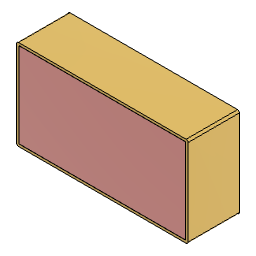
CronusPlastic (Autodesk Fusion 360 design; units mm, degrees)
Autodesk Fusion 360 part; units mm, degrees
note: some values were not read from the file. Chosen so that the rebuilt part matches the saved one: which face or edge a step refers to; which sketch regions a step uses.
sketch "Sketch1" plane through (0, 0, 0) normal (0, 1, 0) x (1, 0, 0) in component "Enclosure"
  line L0 (0, 0) -> (134.4, 0)
  line L1 (134.4, 0) -> (134.4, -70.6)
  line L2 (134.4, -70.6) -> (0, -70.6)
  line L3 (0, -70.6) -> (0, 0)
  dimension "d6" = 134.4
  dimension "d7" = 70.6
  constraint horizontal L0
  constraint vertical L1
  constraint horizontal L2
  constraint vertical L3
  constraint coincident L0.start L3.end
  measures "d6" distance of L0.start L0.end
  measures "d7" distance of L0.start L2.end
extrude "Extrude1" add sketch "Sketch1" along normal blind 40.3 makes body 1 in component "Enclosure"
shell "Shell1" thickness 3 removed faces 1 at (44.8, 0, 23.5333) on bodies 1 in component "Enclosure"
extrude "Extrude2" cut 1 faces at (45.8, 37.3, 24.5333) along direction (0, 1, 0) up to surface (3 mm away) on bodies 1 bodies 1 in component "Enclosure"
ref_plane "WorkPlane1" through (67.2, 2.4, 35.3) normal (0, -1, 0) x (-1, 0, 0) in component "Enclosure"
sketch "Sketch2" plane through (0, 0, 0) normal (0, -1, 0) x (1, 0, 0) in component "Enclosure"
  line L0 (3, 3) -> (3, 67.6)
  line L1 (3, 67.6) -> (131.4, 67.6)
  line L2 (131.4, 67.6) -> (131.4, 3)
  line L3 (131.4, 3) -> (3, 3)
  line L4 (134.4, 70.6) -> (0, 70.6)
  line L5 (0, 70.6) -> (0, 0)
  line L6 (0, 0) -> (134.4, 0)
  line L7 (134.4, 0) -> (134.4, 70.6)
  line L8 (132.4, 2) -> (2, 2)
  line L9 (2, 2) -> (2, 68.6)
  line L10 (2, 68.6) -> (132.4, 68.6)
  line L11 (132.4, 68.6) -> (132.4, 2)
  dimension "d15" = -1
extrude "Extrude3" cut sketch "Sketch2" against normal up to surface (2.4 mm away) contours L8 L9 L10 L11 bodies 1 in component "Enclosure"
sketch "Sketch1 (2)" plane through (0, 2.4, 0) normal (0, -1, 0) x (-1, 0, 0) in component "Display"
  line L0 (-131.4, -67.6) -> (-3, -67.6) construction
  line L1 (-131.4, -3) -> (-131.4, -67.6) construction
  line L2 (-3, -67.6) -> (-3, -3) construction
  line L3 (-3, -3) -> (-131.4, -3) construction
  line L4 (-131.2, -3.2) -> (-131.2, -67.4)
  line L5 (-131.2, -67.4) -> (-3.2, -67.4)
  line L6 (-3.2, -67.4) -> (-3.2, -3.2)
  line L7 (-3.2, -3.2) -> (-131.2, -3.2)
extrude "Extrude1'" add sketch "Sketch1 (2)" against normal blind 12.9 separate body makes body 2 in component "Display"
sketch "Sketch2 (2)" plane through (0, 15.3, 0) normal (0, 1, 0) x (-1, 0, 0) in component "Display"
  line L0 (-131.2, 67.4) -> (-131.2, 61.4) construction
  line L1 (-131.2, 61.4) -> (-3.2, 61.4) construction
  line L2 (-131.2, 61.4) -> (-128.2, 61.4) construction
  circle A0 centre (-128.2, 61.4) radius 1.65
  circle A1 centre (-96.2, 61.4) radius 1.65
  circle A2 centre (-64.2, 61.4) radius 1.65
  circle A3 centre (-32.2, 61.4) radius 1.65
  line L3 (-128.2, 61.4) -> (-102.2, 61.4) construction
  circle A4 centre (-102.2, 61.4) radius 1.65
  circle A5 centre (-70.2, 61.4) radius 1.65
  circle A6 centre (-38.2, 61.4) radius 1.65
  circle A7 centre (-6.2, 61.4) radius 1.65
  circle A8 centre (-128.2, 41.4) radius 1.65
  circle A9 centre (-96.2, 41.4) radius 1.65
  circle A10 centre (-64.2, 41.4) radius 1.65
  circle A11 centre (-32.2, 41.4) radius 1.65
  circle A12 centre (-102.2, 41.4) radius 1.65
  circle A13 centre (-70.2, 41.4) radius 1.65
  circle A14 centre (-38.2, 41.4) radius 1.65
  circle A15 centre (-6.2, 41.4) radius 1.65
  line L4 (-131.2, 35.3) -> (-3.2, 35.3) construction
  circle A16 centre (-128.2, 9.2) radius 1.65
  circle A17 centre (-128.2, 29.2) radius 1.65
  circle A18 centre (-102.2, 29.2) radius 1.65
  circle A19 centre (-102.2, 9.2) radius 1.65
  circle A20 centre (-96.2, 9.2) radius 1.65
  circle A21 centre (-96.2, 29.2) radius 1.65
  circle A22 centre (-70.2, 29.2) radius 1.65
  circle A23 centre (-70.2, 9.2) radius 1.65
  circle A24 centre (-64.2, 9.2) radius 1.65
  circle A25 centre (-64.2, 29.2) radius 1.65
  circle A26 centre (-38.2, 9.2) radius 1.65
  circle A27 centre (-32.2, 9.2) radius 1.65
  circle A28 centre (-38.2, 29.2) radius 1.65
  circle A29 centre (-32.2, 29.2) radius 1.65
  circle A30 centre (-6.2, 9.2) radius 1.65
  circle A31 centre (-6.2, 29.2) radius 1.65
  line L5 (-131.2, 3.2) -> (-3.2, 3.2)
  line L6 (-3.2, 3.2) -> (-3.2, 67.4)
  line L7 (-3.2, 67.4) -> (-131.2, 67.4)
  line L8 (-131.2, 67.4) -> (-131.2, 3.2)
  dimension "d20" = 6
  dimension "d21" = 3
  dimension "d22" = 3.3
  dimension "d25" = 32
  dimension "d26" = -20
  dimension "d27" = 26
  dimension "d28" = 3.3
  dimension "d31" = 32
  dimension "d32" = -20
  constraint perpendicular L0 L2
  constraint coincident L2.end A0.centre
  constraint parallel L1 L3
  constraint coincident L3.end A4.centre
  constraint symmetric A0 L4 A16
  constraint symmetric A1 L4 A20
  constraint symmetric A2 L4 A24
  constraint symmetric A3 L4 A27
  constraint symmetric A4 L4 A19
  constraint symmetric A5 L4 A23
  constraint symmetric A6 L4 A26
  constraint symmetric A7 L4 A30
  constraint symmetric A8 L4 A17
  constraint symmetric A9 L4 A21
  constraint symmetric A10 L4 A25
  constraint symmetric A11 L4 A29
  constraint symmetric A12 L4 A18
  constraint symmetric A13 L4 A22
  constraint symmetric A14 L4 A28
  constraint symmetric A15 L4 A31
  constraint coincident L1.end L6
  constraint coincident L0.end L8
  constraint coincident L0.start L7.end
  constraint midpoint L4.start L8
  constraint midpoint L4.end L6
  measures "d20" distance of L0.end L0.start
  measures "d21" distance of L0.end L2.end
  measures "d22" diameter of A0
  measures "d27" distance of L2.end L3.end
  measures "d28" diameter of A4
extrude "Extrude2'" cut sketch "Sketch2 (2)" against normal blind 2 contours A0 | A1 | A2 | A3 | A4 | A5 | A6 | A7 | A8 | A9 | A10 | A11 | A12 | A13 | A14 | A15 | A16 | A17 | A18 | A19 | A20 | A21 | A22 | A23 | A24 | A25 | A26 | A27 | A28 | A29 | A30 | A31 bodies 2 in component "Display"
sketch "Sketch1 (3)" plane through (0, 15.3, 0) normal (0, 1, 0) x (-1, 0, 0) in component "DisplayMount"
  line L0 (-67.2, 67.4) -> (-67.2, 3.2) construction
  line L1 (-131.2, 3.2) -> (-3.2, 3.2)
  line L2 (-3.2, 3.2) -> (-3.2, 67.4)
  line L3 (-3.2, 67.4) -> (-131.2, 67.4)
  line L4 (-131.2, 67.4) -> (-131.2, 3.2)
  line L5 (-131.2, 67.4) -> (-67.2, 67.4) construction
  line L6 (-99.2, 67.4) -> (-99.2, 3.2) construction
  line L7 (-92.7, 3.2) -> (-105.7, 3.2)
  line L8 (-105.7, 3.2) -> (-105.7, 67.4)
  line L9 (-105.7, 67.4) -> (-92.7, 67.4)
  line L10 (-92.7, 67.4) -> (-92.7, 3.2)
  line L11 (-92.7, 3.2) -> (-105.7, 67.4) construction
  line L12 (-105.7, 3.2) -> (-92.7, 67.4) construction
  line L13 (-28.7, 3.2) -> (-28.7, 67.4)
  line L14 (-28.7, 67.4) -> (-41.7, 67.4)
  line L15 (-41.7, 67.4) -> (-41.7, 3.2)
  line L16 (-41.7, 3.2) -> (-28.7, 3.2)
  line L17 (-105.7, 3.2) -> (-92.7, 3.2)
  line L18 (-92.7, 3.2) -> (-92.7, 6.2)
  line L19 (-92.7, 6.2) -> (-105.7, 6.2)
  line L20 (-105.7, 6.2) -> (-105.7, 3.2)
  line L21 (-41.7, 3.2) -> (-28.7, 3.2)
  line L22 (-28.7, 3.2) -> (-28.7, 6.2)
  line L23 (-28.7, 6.2) -> (-41.7, 6.2)
  line L24 (-41.7, 6.2) -> (-41.7, 3.2)
  circle A0 centre (-96.2, 61.4) radius 1.65
  circle A1 centre (-102.2, 41.4) radius 1.65
  circle A2 centre (-38.2, 61.4) radius 1.65
  circle A3 centre (-32.2, 41.4) radius 1.65
  circle A4 centre (-102.2, 29.2) radius 1.65
  circle A5 centre (-96.2, 9.2) radius 1.65
  circle A6 centre (-32.2, 29.2) radius 1.65
  circle A7 centre (-38.2, 9.2) radius 1.65
  line L25 (-105.7, 67.4) -> (-92.6, 67.4)
  line L26 (-92.6, 67.4) -> (-92.6, 64.4)
  line L27 (-92.6, 64.4) -> (-105.7, 64.4)
  line L28 (-105.7, 64.4) -> (-105.7, 67.4)
  line L29 (-41.7, 67.4) -> (-28.7, 67.4)
  line L30 (-28.7, 67.4) -> (-28.7, 64.4)
  line L31 (-28.7, 64.4) -> (-41.7, 64.4)
  line L32 (-41.7, 64.4) -> (-41.7, 67.4)
  point P0 (-99.2, 35.3)
  dimension "d58" = 13
  dimension "d59" = 3
  dimension "d60" = 3
  dimension "d92" = 3
  dimension "d93" = 3
  constraint midpoint L0.start L3
  constraint midpoint L0.end L1
  constraint coincident L3.end L4.start
  constraint midpoint L5 L6.start
  constraint perpendicular L1 L6
  constraint horizontal L7
  constraint perpendicular L7 L8
  constraint parallel L7 L9
  constraint parallel L8 L10
  constraint coincident L11 P0
  constraint coincident L12 P0
  constraint midpoint L6 P0
  constraint symmetric L0 L7.start L15.end
  constraint symmetric L0 L7.end L13.start
  constraint symmetric L0 L8.end L13.end
  constraint symmetric L0 L9.end L14.end
  constraint horizontal L17
  constraint vertical L18
  constraint horizontal L19
  constraint vertical L20
  constraint coincident L10 L18.end
  constraint horizontal L21
  constraint vertical L22
  constraint horizontal L23
  constraint vertical L24
  constraint coincident L13 L22.end
  constraint collinear L5 L9
  constraint collinear L1 L17
  constraint horizontal L25
  constraint vertical L26
  constraint horizontal L27
  constraint vertical L28
  constraint horizontal L29
  constraint vertical L30
  constraint horizontal L31
  constraint vertical L32
  constraint collinear L13 L30
  measures "d58" distance of L8.end L9.end
  measures "d59" distance of L7.end L19.end
  measures "d60" distance of L15.end L23.end
  measures "d92" distance of L8.end L27.end
  measures "d93" distance of L14.end L31.end
extrude "Extrude1''" add sketch "Sketch1 (3)" along normal blind 3 separate body contours L8 L10 L19 L27 | L3 L8 L9 L10 L25 L27 L28 | L13 L15 L23 L31 | L3 L13 L14 L15 L29 L30 L31 L32 makes body 3 at (101.9708, 15.3, 14.7288) makes body 4 at (32.4292, 15.3, 14.7288) in component "DisplayMount"
extrude "Extrude2''" add sketch "Sketch1 (3)" along normal blind 23.2 contours L1 L7 L8 L10 L17 L18 L19 L20 | L3 L8 L9 L10 L25 L27 L28 | L1 L13 L15 L16 L21 L22 L23 L24 | L3 L13 L14 L15 L29 L30 L31 L32 bodies 3 4 in component "DisplayMount"
chamfer "Chamfer1" distance 4 angle 45 2 edges at (99.2, 18.3, 6.2) (35.2, 18.3, 6.2) on bodies 3 4 in component "DisplayMount"
chamfer "Chamfer1" distance 4 angle 45 2 edges at (99.2, 18.3, 64.4) (35.2, 18.3, 64.4) on bodies 3 4 in component "DisplayMount"
sketch "Sketch3" plane through (0, 18.3, 0) normal (0, 1, 0) x (-1, 0, 0) in component "DisplayMount"
  line L0 (-105.7, 10.2) -> (-28.6, 67.9) construction
  line L1 (-67.15, 39.05) -> (-67.15, 35.65) construction
  line L2 (-34.15, 12.65) -> (-100.15, 12.65) construction
  line L3 (-100.15, 12.65) -> (-100.15, 58.65) construction
  line L4 (-100.15, 58.65) -> (-34.15, 58.65) construction
  line L5 (-34.15, 58.65) -> (-34.15, 12.65) construction
  line L6 (-34.15, 12.65) -> (-100.15, 58.65) construction
  line L7 (-100.15, 12.65) -> (-34.15, 58.65) construction
  circle A0 centre (-100.15, 58.65) radius 1
  circle A1 centre (-100.15, 58.65) radius 2.15
  circle A2 centre (-34.15, 58.65) radius 2.15
  circle A3 centre (-34.15, 58.65) radius 1
  circle A4 centre (-100.15, 12.65) radius 2.15
  circle A5 centre (-100.15, 12.65) radius 1
  circle A6 centre (-34.15, 12.65) radius 2.15
  circle A7 centre (-34.15, 12.65) radius 1
  circle A8 centre (-96.2, 61.4) radius 3
  circle A9 centre (-38.2, 61.4) radius 3
  circle A10 centre (-96.2, 9.2) radius 1.65
  circle A11 centre (-38.2, 9.2) radius 1.65
  circle A12 centre (-96.2, 9.2) radius 3
  circle A13 centre (-38.2, 9.2) radius 3
  arc A14 (-97.5124, 60.4) -> (-94.8876, 60.4) centre (-96.2, 61.4) ccw
  arc A15 (-39.5124, 60.4) -> (-36.8876, 60.4) centre (-38.2, 61.4) ccw
  point P0 (-105.7, 10.2)
  point P1 (-28.7, 67.4)
  dimension "d65" = 3.4
  dimension "d66" = 66
  dimension "d67" = 46
  dimension "d70" = 2
  dimension "d71" = 4.3
  dimension "d74" = 66
  dimension "d75" = -46
  dimension "d76" = 6
  dimension "d77" = 6
  dimension "d89" = 6
  dimension "d90" = 6
  constraint coincident P0 L0.start
  constraint vertical L1
  constraint midpoint L0 L1.start
  constraint horizontal L2
  constraint perpendicular L2 L3
  constraint parallel L2 L4
  constraint parallel L3 L5
  constraint coincident L3.end L4.start
  constraint concentric A0 A1
  constraint concentric A8 A14
  constraint concentric A9 A15
  constraint concentric A10 A12
  constraint concentric A11 A13
  constraint midpoint L1.end L7
  measures "d65" distance of L1.start L1.end
  measures "d66" distance of L3.end L4.end
  measures "d67" distance of L2.end L3.end
  measures "d70" diameter of A0
  measures "d71" diameter of A1
  measures "d76" diameter of A8
  measures "d77" diameter of A9
  measures "d89" diameter of A12
  measures "d90" diameter of A13
extrude "Extrude5" add sketch "Sketch3" along normal blind 4 contours A1 A8 | A1 A8 | A2 A9 | A2 A9 | A4 | A6 picked at (-99.3568, 60.1302) picked at (-98.5668, 59.7522) picked at (-35.7986, 59.0039) picked at (-35.8985, 59.6123) bodies 3 4 in component "DisplayMount"
chamfer "Chamfer2" distance 2 angle 45 4 edges at (100.15, 18.3, 56.5) (102.1545, 18.3, 13.4275) (34.15, 18.3, 56.5) (36.1545, 18.3, 13.4275) on bodies 3 4 in component "DisplayMount"
extrude "Extrude6" cut sketch "Sketch3" along normal up to surface (20.2 mm away) contours A1 A8 | A2 A9 | A12 | A13 picked at (-95.3701, 62.1374) picked at (-39.1425, 61.9294) bodies 3 4 in component "DisplayMount"
extrude "Extrude7" cut sketch "Sketch3" along normal up to surface (20.2 mm away) contours A1 A8 | A1 A8 | A2 A9 | A2 A9 | A3 | A12 | A13 picked at (-98.5668, 59.7522) picked at (-95.3701, 62.1374) picked at (-35.8985, 59.6123) picked at (-39.1425, 61.9294) bodies 3 4 in component "DisplayMount"
extrude "Extrude8" cut sketch "Sketch3" against normal up to surface (3 mm away) contours A0 | A3 | A5 | A7 bodies 3 4 in component "DisplayMount"
sketch "Sketch4" plane through (0, 38.5, 0) normal (0, 1, 0) x (-1, 0, 0) in component "DisplayMount"
  line L0 (-105.7, 67.4) -> (-102.518, 64.218) construction
  line L1 (-105.7, 67.4) -> (-99.6, 67.4) construction
  circle A0 centre (-102.518, 64.218) radius 1.5
  circle A1 centre (-102.518, 64.218) radius 2.95
  line L2 (-92.7, 67.4) -> (-41.7, 67.4) construction
  line L3 (-92.7, 3.2) -> (-41.7, 3.2) construction
  line L4 (-67.2, 67.4) -> (-67.2, 3.2) construction
  line L5 (-67.2, 35.3) -> (-57.2, 35.3) construction
  circle A2 centre (-31.882, 64.218) radius 2.95
  circle A3 centre (-31.882, 64.218) radius 1.5
  circle A4 centre (-102.518, 6.382) radius 2.95
  circle A5 centre (-102.518, 6.382) radius 1.5
  circle A6 centre (-31.882, 6.382) radius 2.95
  circle A7 centre (-31.882, 6.382) radius 1.5
  point P0 (-105.7, 67.4)
  point P1 (-92.7, 67.4)
  point P2 (-41.7, 67.4)
  point P3 (-92.7, 3.2)
  point P4 (-41.7, 3.2)
  dimension "d95" = 45
  dimension "d96" = 4.5
  dimension "d97" = 3
  dimension "d98" = 10
  dimension "d220" = 5.9
  constraint horizontal L1
  constraint coincident P0 L0.start
  constraint coincident L0.end A0.centre
  constraint concentric A0 A1
  constraint coincident P1 L2.start
  constraint coincident P2 L2.end
  constraint coincident P3 L3.start
  constraint coincident P4 L3.end
  constraint midpoint L2 L4.start
  constraint midpoint L3 L4.end
  constraint horizontal L5
  constraint midpoint L4 L5.start
  constraint symmetric A0 L4 A3
  constraint symmetric A1 L4 A2
  constraint symmetric A0 L5 A5
  constraint symmetric A1 L5 A4
  constraint symmetric L5 A2 A6
  constraint symmetric L5 A3 A7
  measures "d95" angle of L0 L1
  measures "d96" distance of P0 L0.end
  measures "d97" diameter of A0
  measures "d98" distance of L5.start L5.end
  measures "d220" diameter of A1
extrude "Extrude9" add sketch "Sketch4" against normal up to surface (23.2 mm away) bodies 3 4 in component "DisplayMount"
extrude "Extrude10" cut sketch "Sketch4" against normal up to surface (20.2 mm away) contours A0 | A3 | A5 | A7 bodies 3 4 in component "DisplayMount"
ref_plane "WorkPlane2" through (67.2, 38.5, 35.3) normal (0, 1, 0) x (0, 0, 1) in component "Enclosure"
sketch "Sketch5" plane through (0, 38.5, 0) normal (0, 1, 0) x (1, 0, 0) in component "Enclosure"
  line L0 (131.4, -3) -> (131.4, -67.6) construction
  line L1 (131.4, -67.6) -> (3, -67.6) construction
  line L2 (3, -3) -> (131.4, -3) construction
  line L3 (3, -67.6) -> (3, -3) construction
  line L4 (67.2, -67.6) -> (67.2, -3) construction
  line L5 (131.4, -35.3) -> (3, -35.3) construction
  line L6 (131.4, -3) -> (3, -3)
  line L7 (131.4, -3) -> (140.1172, -3) construction
  line L8 (129.9, -32.3) -> (132.9, -32.3)
  line L9 (132.9, -32.3) -> (132.9, -38.3)
  line L10 (132.9, -38.3) -> (129.9, -38.3)
  line L11 (129.9, -38.3) -> (129.9, -32.3)
  line L12 (129.9, -32.3) -> (132.9, -38.3) construction
  line L13 (132.9, -32.3) -> (129.9, -38.3) construction
  line L14 (1.5, -38.3) -> (4.5, -38.3)
  line L15 (4.5, -38.3) -> (4.5, -32.3)
  line L16 (4.5, -32.3) -> (1.5, -32.3)
  line L17 (131.4, -3) -> (131.4, -67.6)
  line L18 (131.4, -67.6) -> (3, -67.6)
  line L19 (3, -67.6) -> (3, -3)
  line L20 (3, -3) -> (131.4, -3)
  line L21 (0, -70.6) -> (134.4, -70.6)
  line L22 (134.4, -70.6) -> (134.4, 0)
  line L23 (134.4, 0) -> (0, 0)
  line L24 (0, 0) -> (0, -70.6)
  line L25 (131.4, -67.6) -> (126.4, -67.6)
  line L26 (126.4, -67.6) -> (126.4, -62.6)
  line L27 (126.4, -62.6) -> (131.4, -62.6)
  line L28 (131.4, -62.6) -> (131.4, -67.6)
  line L29 (126.4, -62.6) -> (131.4, -67.6) construction
  circle A0 centre (128.9, -65.1) radius 1.4
  line L30 (3, -67.6) -> (8, -67.6)
  line L31 (3, -62.6) -> (3, -67.6)
  circle A1 centre (5.5, -65.1) radius 1.4
  line L32 (8, -62.6) -> (3, -62.6)
  line L33 (8, -67.6) -> (8, -62.6)
  line L34 (126.4, -3) -> (126.4, -8)
  line L35 (126.4, -8) -> (131.4, -8)
  circle A2 centre (128.9, -5.5) radius 1.4
  line L36 (131.4, -8) -> (131.4, -3)
  line L37 (131.4, -3) -> (126.4, -3)
  line L38 (8, -3) -> (8, -8)
  line L39 (3, -3) -> (8, -3)
  circle A3 centre (5.5, -5.5) radius 1.4
  line L40 (8, -8) -> (3, -8)
  line L41 (3, -8) -> (3, -3)
  line L42 (105.7, -67.4) -> (105.7, -64.4) construction
  line L43 (92.7, -64.4) -> (92.7, -67.4) construction
  line L44 (131.4, -67.6) -> (3, -67.6) construction
  line L45 (108.7, -67.6) -> (105.7, -67.6)
  line L46 (105.7, -67.6) -> (105.7, -64.6)
  line L47 (105.7, -64.6) -> (108.7, -64.6)
  line L48 (108.7, -64.6) -> (108.7, -67.6)
  line L49 (92.7, -67.6) -> (89.7, -67.6)
  line L50 (89.7, -67.6) -> (89.7, -64.6)
  line L51 (89.7, -64.6) -> (92.7, -64.6)
  line L52 (92.7, -64.6) -> (92.7, -67.6)
  line L53 (25.7, -64.6) -> (25.7, -67.6)
  line L54 (25.7, -67.6) -> (28.7, -67.6)
  line L55 (28.7, -64.6) -> (25.7, -64.6)
  line L56 (28.7, -67.6) -> (28.7, -64.6)
  line L57 (44.7, -64.6) -> (41.7, -64.6)
  line L58 (41.7, -64.6) -> (41.7, -67.6)
  line L59 (44.7, -67.6) -> (44.7, -64.6)
  line L60 (41.7, -67.6) -> (44.7, -67.6)
  line L61 (105.7, -6) -> (108.7, -6)
  line L62 (108.7, -6) -> (108.7, -3)
  line L63 (108.7, -3) -> (105.7, -3)
  line L64 (105.7, -3) -> (105.7, -6)
  line L65 (92.7, -6) -> (92.7, -3)
  line L66 (89.7, -6) -> (92.7, -6)
  line L67 (89.7, -3) -> (89.7, -6)
  line L68 (92.7, -3) -> (89.7, -3)
  line L69 (44.7, -6) -> (41.7, -6)
  line L70 (44.7, -3) -> (44.7, -6)
  line L71 (41.7, -6) -> (41.7, -3)
  line L72 (41.7, -3) -> (44.7, -3)
  line L73 (28.7, -3) -> (28.7, -6)
  line L74 (25.7, -3) -> (28.7, -3)
  line L75 (28.7, -6) -> (25.7, -6)
  line L76 (25.7, -6) -> (25.7, -3)
  point P0 (131.4, -35.3)
  dimension "d110" = 3
  dimension "d111" = 6
  dimension "d183" = 5
  dimension "d184" = 5
  dimension "d185" = 2.8
  dimension "d199" = 3
  dimension "d200" = 3
  dimension "d201" = 3
  dimension "d202" = 3
  constraint midpoint L2 L4.end
  constraint midpoint L0 P0
  constraint midpoint L3 L5.end
  constraint horizontal L8
  constraint perpendicular L8 L9
  constraint parallel L8 L10
  constraint parallel L9 L11
  constraint coincident L12 P0
  constraint coincident L13 P0
  constraint coincident P0 L5.start
  constraint symmetric L4 L8.start L15.end
  constraint symmetric L4 L8.end L16.end
  constraint symmetric L4 L9.end L14.start
  constraint symmetric L4 L10.end L14.end
  constraint midpoint L1 L4.start
  constraint horizontal L25
  constraint vertical L26
  constraint horizontal L27
  constraint vertical L28
  constraint coincident L0.end L1.start
  constraint midpoint L29 A0.centre
  constraint symmetric L4 L0.end L1.end
  constraint symmetric L4 L25.end L30.end
  constraint symmetric L4 L26.end L32.start
  constraint symmetric L4 L27.end L31.start
  constraint symmetric L4 A0 A1
  constraint symmetric L5 L0.end L0.start
  constraint symmetric L5 L25.end L34.start
  constraint symmetric L5 L26.end L34.end
  constraint symmetric L5 L27.end L35.end
  constraint symmetric L5 A0 A2
  constraint symmetric L5 L1.end L2.start
  constraint symmetric L5 L30.end L38.start
  constraint symmetric L5 L31.start L40.end
  constraint symmetric L5 A1 A3
  constraint symmetric L5 L32.start L38.end
  constraint horizontal L45
  constraint vertical L46
  constraint horizontal L47
  constraint vertical L48
  constraint coincident L44 L45.start
  constraint collinear L42 L46
  constraint horizontal L49
  constraint vertical L50
  constraint horizontal L51
  constraint vertical L52
  constraint coincident L44 L49.start
  constraint collinear L43 L52
  constraint symmetric L4 L45.start L53.end
  constraint symmetric L4 L45.end L54.end
  constraint symmetric L4 L46.end L55.start
  constraint symmetric L4 L47.end L53.start
  constraint symmetric L4 L49.start L58.end
  constraint symmetric L4 L49.end L59.start
  constraint symmetric L4 L50.end L57.start
  constraint symmetric L4 L51.end L57.end
  constraint symmetric L5 L45.start L62.end
  constraint symmetric L5 L45.end L63.end
  constraint symmetric L5 L46.end L61.start
  constraint symmetric L5 L47.end L61.end
  constraint symmetric L5 L49.start L65.end
  constraint symmetric L5 L49.end L67.start
  constraint symmetric L5 L50.end L66.start
  constraint symmetric L5 L51.end L65.start
  constraint symmetric L5 L53.start L75.end
  constraint symmetric L5 L53.end L74.start
  constraint symmetric L5 L54.end L73.start
  constraint symmetric L5 L55.start L73.end
  constraint symmetric L5 L57.start L69.start
  constraint symmetric L5 L57.end L69.end
  constraint symmetric L5 L58.end L71.end
  constraint symmetric L5 L59.start L70.start
  measures "d110" distance of L9.end L10.end
  measures "d111" distance of L8.end L9.end
  measures "d183" distance of L0.end L25.end
  measures "d184" distance of L0.end L27.end
  measures "d185" diameter of A0
  measures "d199" distance of L45.start L45.end
  measures "d200" distance of L45.start L47.end
  measures "d201" distance of L49.start L49.end
  measures "d202" distance of L49.start L51.end
extrude "Extrude8'" add sketch "Sketch5" against normal blind 10 contours L6 L17 L20 L34 L35 L36 L37 | L17 L18 L25 L26 L27 L28 | L6 L19 L20 L38 L39 L40 L41 | L18 L19 L30 L31 L32 L33 | A0 | A1 | A2 | A3 bodies 1 in component "Enclosure"
extrude "Extrude19" add sketch "Sketch5" against normal blind 3 contours L8 L10 L11 L17 | L14 L15 L16 L19 bodies 1 in component "Enclosure"
extrude "Extrude14" cut sketch "Sketch5" against normal up to surface (9 mm away) contours A0 | A1 | A2 | A3 bodies 1 in component "Enclosure"
chamfer "Chamfer6" distance 4.9 angle 45 6 edges at (128.9, 28.5, 3) (128.9, 28.5, 67.6) (5.5, 28.5, 67.6) (5.5, 28.5, 67.6) (5.5, 28.5, 3) (128.9, 28.5, 3) on bodies 1 in component "Enclosure"
chamfer "Chamfer9" distance 1.5 angle 45 2 edges at (131.4, 35.5, 35.3) (3, 35.5, 35.3) on bodies 1 in component "Enclosure"
extrude "Extrude20" add sketch "Sketch5" against normal up to surface (23.2 mm away) contours L6 L20 L61 L62 L63 L64 | L6 L20 L65 L66 L67 L68 | L6 L20 L69 L70 L71 L72 | L18 L45 L46 L47 L48 | L6 L20 L73 L74 L75 L76 | L18 L49 L50 L51 L52 | L18 L57 L58 L59 L60 | L18 L53 L54 L55 L56 bodies 1 in component "Enclosure"
chamfer "Chamfer10" distance 3 angle 45 4 edges at (27.2, 15.3, 6) (43.2, 15.3, 6) (91.2, 15.3, 6) (107.2, 15.3, 6) on bodies 1 in component "Enclosure"
chamfer "Chamfer10" distance 3 angle 45 4 edges at (27.2, 15.3, 64.6) (43.2, 15.3, 64.6) (91.2, 15.3, 64.6) (107.2, 15.3, 64.6) on bodies 1 in component "Enclosure"
sketch "Sketch7" plane through (0, 0, 3) normal (0, 0, 1) x (-1, 0, 0) in component "Enclosure"
  line L0 (-131.4, -2.4) -> (-131.4, -23.6)
  line L1 (-131.4, -40.3) -> (-3, -40.3)
  line L2 (-105.7, -15.3) -> (-105.7, -38.5)
  line L3 (-92.7, -15.3) -> (-92.7, -38.5)
  line L4 (-41.7, -15.3) -> (-41.7, -38.5)
  line L5 (-28.7, -15.3) -> (-28.7, -38.5)
  line L6 (-105.7, -15.3) -> (-108.7, -15.3)
  line L7 (-108.7, -15.3) -> (-108.7, -38.5)
  line L8 (-108.7, -38.5) -> (-105.7, -38.5)
  line L9 (-105.7, -38.5) -> (-105.7, -15.3)
  line L10 (-92.7, -15.3) -> (-89.7, -15.3)
  line L11 (-89.7, -15.3) -> (-89.7, -38.5)
  line L12 (-89.7, -38.5) -> (-92.7, -38.5)
  line L13 (-92.7, -38.5) -> (-92.7, -15.3)
  line L14 (-41.7, -15.3) -> (-44.7, -15.3)
  line L15 (-44.7, -15.3) -> (-44.7, -38.5)
  line L16 (-44.7, -38.5) -> (-41.7, -38.5)
  line L17 (-41.7, -38.5) -> (-41.7, -15.3)
  line L18 (-28.7, -15.3) -> (-25.7, -15.3)
  line L19 (-25.7, -15.3) -> (-25.7, -38.5)
  line L20 (-25.7, -38.5) -> (-28.7, -38.5)
  line L21 (-28.7, -38.5) -> (-28.7, -15.3)
  line L22 (-3, -23.6) -> (-3, -2.4)
  line L23 (-126.4, -38.5) -> (-131.4, -38.5)
  line L24 (-8, -23.6) -> (-3, -23.6)
  line L25 (-3, -2.4) -> (-131.4, -2.4)
  line L26 (-131.4, -23.6) -> (-126.4, -23.6)
  line L27 (-126.4, -23.6) -> (-126.4, -38.5)
  line L28 (-8, -38.5) -> (-8, -23.6)
  line L29 (-28.7, -38.5) -> (-28.7, -15.3)
  line L30 (-28.7, -15.3) -> (-25.7, -15.3)
  line L31 (-25.7, -15.3) -> (-25.7, -38.5)
  line L32 (-25.7, -38.5) -> (-28.7, -38.5)
  line L33 (-108.7, -38.5) -> (-108.7, -15.3)
  line L34 (-108.7, -15.3) -> (-105.7, -15.3)
  line L35 (-105.7, -15.3) -> (-105.7, -38.5)
  line L36 (-105.7, -38.5) -> (-108.7, -38.5)
  line L37 (-44.7, -38.5) -> (-44.7, -15.3)
  line L38 (-44.7, -15.3) -> (-41.7, -15.3)
  line L39 (-41.7, -15.3) -> (-41.7, -38.5)
  line L40 (-41.7, -38.5) -> (-44.7, -38.5)
  line L41 (-89.7, -15.3) -> (-89.7, -38.5)
  line L42 (-89.7, -38.5) -> (-92.7, -38.5)
  line L43 (-92.7, -38.5) -> (-92.7, -15.3)
  line L44 (-92.7, -15.3) -> (-89.7, -15.3)
  line L45 (-131.4, -38.5) -> (-131.4, -40.3)
  line L46 (-3, -40.3) -> (-3, -38.5)
  line L47 (-3, -38.5) -> (-8, -38.5)
  dimension "d123" = 3
  dimension "d124" = 3
  dimension "d125" = 3
  dimension "d126" = 3
  constraint horizontal L6
  constraint vertical L7
  constraint horizontal L8
  constraint vertical L9
  constraint coincident L2.start L6.start
  constraint horizontal L10
  constraint vertical L11
  constraint horizontal L12
  constraint vertical L13
  constraint coincident L3.start L10.start
  constraint horizontal L14
  constraint vertical L15
  constraint horizontal L16
  constraint vertical L17
  constraint coincident L4.start L14.start
  constraint horizontal L18
  constraint vertical L19
  constraint horizontal L20
  constraint vertical L21
  constraint coincident L5.start L18.start
  constraint coincident L2.end L8.end
  constraint coincident L3.end L12.end
  constraint coincident L4.end L16.end
  constraint coincident L5.end L20.end
  measures "d123" distance of L2.start L6.end
  measures "d124" distance of L3.start L10.end
  measures "d125" distance of L4.start L14.end
  measures "d126" distance of L5.start L18.end
extrude "Extrude11" add sketch "Sketch7" along normal blind 3 contours L2 L6 L7 L8 L9 L33 L34 L35 L36 | L3 L10 L11 L12 L13 L41 L42 L43 L44 | L4 L14 L15 L16 L17 L37 L38 L39 L40 | L5 L18 L19 L20 L21 L29 L30 L31 L32 bodies 1 in component "Enclosure"
chamfer "Chamfer2'" distance 3 angle 45 4 edges at (107.2, 15.3, 6) (91.2, 15.3, 6) (43.2, 15.3, 6) (27.2, 15.3, 6) on bodies 1 in component "Enclosure"
sketch "Sketch8" plane through (0, 0, 3) normal (0, 0, 1) x (-1, 0, 0) in component "Enclosure"
  line L0 (-89.7, -38.5) -> (-44.7, -38.5) construction
  line L1 (-67.2, -38.5) -> (-67.2, -24.5) construction
  line L2 (-57, -38.5) -> (-77.4, -38.5)
  line L3 (-77.4, -38.5) -> (-77.4, -24.5)
  line L4 (-77.4, -24.5) -> (-57, -24.5)
  line L5 (-57, -24.5) -> (-57, -38.5)
  line L6 (-57, -38.5) -> (-77.4, -24.5) construction
  line L7 (-77.4, -38.5) -> (-57, -24.5) construction
  line L8 (-78.4, -38.5) -> (-78.4, -23.5)
  line L9 (-78.4, -23.5) -> (-56, -23.5)
  line L10 (-56, -23.5) -> (-56, -38.5)
  line L11 (-78.4, -38.5) -> (-77.4, -38.5)
  line L12 (-56, -38.5) -> (-57, -38.5)
  point P0 (-44.7, -38.5)
  point P1 (-67.2, -31.5)
  point P2 (-89.7, -38.5)
  dimension "d131" = 14
  dimension "d132" = 20.4
  dimension "d133" = 14
  dimension "d134" = -1
  constraint coincident P0 L0.end
  constraint vertical L1
  constraint midpoint L0 L1.start
  constraint horizontal L2
  constraint perpendicular L2 L3
  constraint parallel L2 L4
  constraint parallel L3 L5
  constraint coincident L6 P1
  constraint coincident L7 P1
  constraint midpoint L1 P1
  constraint perpendicular L3 L11
  constraint perpendicular L5 L12
  measures "d131" distance of L1.start L1.end
  measures "d132" distance of L3.end L4.end
  measures "d133" distance of L2.end L3.end
chamfer "Chamfer8" distance 1.5 angle 45 4 edges at (131.4, 28.5, 7.95) (131.4, 28.5, 62.65) (3, 28.5, 62.65) (3, 28.5, 7.95) on bodies 1 in component "Enclosure"
extrude "Extrude12" add sketch "Sketch8" along normal blind 3 contours L2 L3 L4 L5 bodies 1 in component "Enclosure"
extrude "Extrude13" add sketch "Sketch8" along normal blind 4.6 contours L3 L4 L5 L8 L9 L10 L11 L12 bodies 1 in component "Enclosure"
chamfer "Chamfer4" distance 4 angle 45 1 edges at (67.2, 23.5, 3) on bodies 1 in component "Enclosure"
chamfer "Chamfer5" distance 0.5 angle 45 1 edges at (67.2, 23.5, 7.6) on bodies 1 in component "Enclosure"
sketch "Sketch1 (4)" plane through (0, 0, 6) normal (0, 0, 1) x (-1, 0, 0) in component "PwrBoard"
  line L0 (-57, -24.5) -> (-77.4, -24.5)
  line L1 (-77.4, -24.5) -> (-77.4, -38.5)
  line L2 (-77.4, -38.5) -> (-57, -38.5)
  line L3 (-57, -38.5) -> (-57, -24.5)
  line L4 (-77.4, -24.5) -> (-57, -24.5)
  line L5 (-57, -24.5) -> (-57, -38.5)
  line L6 (-57, -38.5) -> (-77.4, -38.5)
  line L7 (-77.4, -38.5) -> (-77.4, -24.5)
  line L8 (-77.4, -38.5) -> (-74.8997, -35.9997) construction
  line L9 (-77.4, -38.5) -> (-73.764, -38.5) construction
  line L10 (-57, -38.5) -> (-59.5003, -35.9997) construction
  line L11 (-57, -38.5) -> (-60.436, -38.5) construction
  circle A0 centre (-74.8997, -35.9997) radius 0.75
  circle A1 centre (-59.5003, -35.9997) radius 0.75
  dimension "d144" = 3.536
  dimension "d145" = 45
  dimension "d146" = 45
  dimension "d147" = 3.536
  dimension "d148" = 1.5
  dimension "d149" = 1.5
  constraint horizontal L4
  constraint vertical L5
  constraint horizontal L6
  constraint vertical L7
  constraint coincident L2.end L3.start
  constraint coincident L0.end L1.start
  constraint horizontal L9
  constraint coincident L1.end L2.start
  constraint horizontal L11
  constraint coincident L8.end A0.centre
  constraint coincident L10.end A1.centre
  measures "d144" distance of L1.end L8.end
  measures "d145" angle of L8 L9
  measures "d146" angle of L10 L11
  measures "d147" distance of L2.end L10.end
  measures "d148" diameter of A0
  measures "d149" diameter of A1
extrude "Extrude1'''" add sketch "Sketch1 (4)" along normal blind 1.6 separate body makes body 5 in component "PwrBoard"
sketch "Sketch2 (3)" plane through (0, 0, 7.6) normal (0, 0, 1) x (-1, 0, 0) in component "PwrBoard"
  circle A0 centre (-59.5003, -35.9997) radius 0.75
  circle A1 centre (-74.8997, -35.9997) radius 0.75
  line L0 (-77.4, -38.5) -> (-57, -38.5)
  line L1 (-57, -38.5) -> (-57, -24.5)
  line L2 (-57, -24.5) -> (-77.4, -24.5)
  line L3 (-77.4, -24.5) -> (-77.4, -38.5)
  line L4 (-67.2, -38.5) -> (-71.7, -38.5) construction
  line L5 (-67.2, -38.5) -> (-67.2, -31) construction
  line L6 (-67.2, -31) -> (-62.7, -31) construction
  line L7 (-71.7, -38.5) -> (-62.7, -38.5)
  line L8 (-62.7, -38.5) -> (-62.7, -31)
  line L9 (-62.7, -31) -> (-71.7, -31)
  line L10 (-71.7, -31) -> (-71.7, -38.5)
  dimension "d152" = 4.5
  dimension "d153" = 7.5
  dimension "d154" = 4.5
  constraint midpoint L0 L4.start
  constraint horizontal L4
  constraint vertical L5
  constraint horizontal L6
  constraint horizontal L7
  constraint vertical L8
  constraint horizontal L9
  constraint vertical L10
  measures "d152" distance of L4.start L4.end
  measures "d153" distance of L4.start L5.end
  measures "d154" distance of L5.end L6.end
extrude "Extrude2'''" add sketch "Sketch2 (3)" along normal blind 3.2 separate body contours L0 L7 L8 L9 L10 makes body 6 in component "PwrBoard"
fillet "Fillet1" radius 1 4 edges at (71.7, 34.75, 10.8) (71.7, 34.75, 7.6) (62.7, 34.75, 7.6) (62.7, 34.75, 10.8) on bodies 6 in component "PwrBoard"
sketch "Sketch1 (5)" plane through (0, 40.3, 0) normal (0, 1, 0) x (-1, 0, 0) in component "LightSensor"
  line L0 (-131.4, 3) -> (-131.4, 67.6)
  line L1 (-131.4, 67.6) -> (-3, 67.6) construction
  line L2 (-3, 67.6) -> (-3, 3)
  line L3 (-3, 3) -> (-131.4, 3)
  line L4 (0, 70.6) -> (-134.4, 70.6)
  line L5 (-134.4, 70.6) -> (-134.4, 0)
  line L6 (-134.4, 0) -> (0, 0)
  line L7 (0, 0) -> (0, 70.6)
  line L8 (-131.4, 67.6) -> (-3, 67.6)
  line L9 (-69.675, 67.6) -> (-64.725, 67.6) construction
  line L10 (-64.725, 67.6) -> (-64.725, 60.6) construction
  line L11 (-64.725, 60.6) -> (-69.675, 60.6) construction
  line L12 (-69.675, 60.6) -> (-69.675, 67.6) construction
  line L13 (-68.425, 60.6) -> (-65.975, 60.6)
  line L14 (-64.725, 61.85) -> (-64.725, 63.35)
  line L15 (-65.975, 64.6) -> (-68.425, 64.6)
  line L16 (-69.675, 63.35) -> (-69.675, 61.85)
  arc A0 (-68.425, 64.6) -> (-69.675, 63.35) centre (-68.425, 63.35) ccw
  arc A1 (-69.675, 61.85) -> (-68.425, 60.6) centre (-68.425, 61.85) ccw
  arc A2 (-65.975, 60.6) -> (-64.725, 61.85) centre (-65.975, 61.85) ccw
  arc A3 (-64.725, 63.35) -> (-65.975, 64.6) centre (-65.975, 63.35) ccw
  point P0 (-69.675, 64.6)
  dimension "d159" = 4.95
  dimension "d160" = 7
  dimension "d161" = 4
  dimension "d162" = 1.25
  dimension "d163" = 1.25
  dimension "d164" = 1.25
  dimension "d165" = 1.25
  constraint horizontal L9
  constraint vertical L10
  constraint horizontal L11
  constraint vertical L12
  constraint coincident L8 L9.start
  constraint midpoint L8 L9
  constraint horizontal L13
  constraint vertical L14
  constraint horizontal L15
  constraint vertical L16
  constraint coincident P0 L15
  constraint coincident P0 L16
  constraint tangent L15 A0
  constraint tangent L16 A0
  constraint coincident L11.end L13
  constraint coincident L11.end L16
  constraint tangent L13 A1
  constraint tangent L16 A1
  constraint tangent L13 A2
  constraint tangent L14 A2
  constraint tangent L15 A3
  constraint tangent L14 A3
  measures "d159" distance of L9.start L9.end
  measures "d160" distance of L9.start L11.end
  measures "d161" distance of L11.end P0
  measures "d162" radius of A0
  measures "d163" radius of A1
  measures "d164" radius of A2
  measures "d165" radius of A3
extrude "Extrude1''''" add sketch "Sketch1 (5)" against normal blind 1.9 separate body contours L13 L14 L15 L16 A0 A1 A2 A3 makes body 7 in component "LightSensor"
sketch "Sketch9" plane through (0, 38.5, 0) normal (0, 1, 0) x (1, 0, 0) in component "Enclosure"
  arc A0 (64.725, -63.35) -> (65.975, -64.6) centre (65.975, -63.35) ccw construction
  line L0 (65.975, -64.6) -> (68.425, -64.6) construction
  arc A1 (68.425, -64.6) -> (69.675, -63.35) centre (68.425, -63.35) ccw construction
  line L1 (69.675, -63.35) -> (69.675, -61.85) construction
  arc A2 (69.675, -61.85) -> (68.425, -60.6) centre (68.425, -61.85) ccw construction
  line L2 (68.425, -60.6) -> (65.975, -60.6) construction
  arc A3 (65.975, -60.6) -> (64.725, -61.85) centre (65.975, -61.85) ccw construction
  line L3 (64.725, -61.85) -> (64.725, -63.35) construction
  line L4 (65.975, -64.8) -> (68.425, -64.8)
  arc A4 (68.425, -64.8) -> (69.875, -63.35) centre (68.425, -63.35) ccw
  line L5 (69.875, -63.35) -> (69.875, -61.85)
  arc A5 (69.875, -61.85) -> (68.425, -60.4) centre (68.425, -61.85) ccw
  line L6 (68.425, -60.4) -> (65.975, -60.4)
  arc A6 (65.975, -60.4) -> (64.525, -61.85) centre (65.975, -61.85) ccw
  line L7 (64.525, -61.85) -> (64.525, -63.35)
  arc A7 (64.525, -63.35) -> (65.975, -64.8) centre (65.975, -63.35) ccw
  line L8 (71.675, -67.6) -> (62.725, -67.6)
  line L9 (62.725, -67.6) -> (62.725, -58.6)
  line L10 (62.725, -58.6) -> (71.675, -58.6)
  line L11 (71.675, -58.6) -> (71.675, -67.6)
  line L12 (131.4, -67.6) -> (3, -67.6)
  line L13 (69.875, -63.1) -> (64.525, -63.1)
  line L14 (64.525, -63.1) -> (64.525, -62.1)
  line L15 (64.525, -62.1) -> (69.875, -62.1)
  line L16 (69.875, -62.1) -> (69.875, -63.1)
  dimension "d168" = 0.2
  dimension "d169" = 8.95
  dimension "d170" = 9
  dimension "d176" = 1
  constraint horizontal L8
  constraint vertical L9
  constraint horizontal L10
  constraint vertical L11
  constraint midpoint L8 L12
  constraint horizontal L13
  constraint vertical L14
  constraint horizontal L15
  constraint vertical L16
  constraint coincident L5 L13.start
  constraint midpoint L5 L16
  measures "d169" distance of L8.start L8.end
  measures "d170" distance of L8.start L10.end
  measures "d176" distance of L13.start L15.end
extrude "Extrude15" add sketch "Sketch9" against normal blind 3 contours L4 A4 L5 L7 A7 L13 | L5 L7 L13 L14 L15 L16 | L5 A5 L6 A6 L7 L15 | L8 L9 L10 L11 L12 bodies 1 in component "Enclosure"
extrude "Extrude16" cut sketch "Sketch9" against normal blind 0.2 contours L4 A4 L5 L7 A7 L13 | L5 L7 L13 L14 L15 L16 | L5 A5 L6 A6 L7 L15 bodies 1 in component "Enclosure"
chamfer "Chamfer7" distance 9 angle 45 1 edges at (67.2, 35.5, 67.6) on bodies 1 in component "Enclosure"
extrude "Extrude17" cut sketch "Sketch9" along normal up to surface contours L5 L7 L13 L14 L15 L16 end surface through (71.675, 31.0009, 63.1009) normal (0, -0.707107, -0.707107) offset 0 bodies 1 in component "Enclosure"
sketch "Sketch10" plane through (0, 0, 6) normal (0, 0, 1) x (-1, 0, 0) in component "Enclosure"
  line L0 (-57, -24.5) -> (-77.4, -24.5)
  line L1 (-77.4, -24.5) -> (-77.4, -38.5)
  line L2 (-77.4, -38.5) -> (-57, -38.5)
  line L3 (-57, -38.5) -> (-57, -24.5)
  circle A0 centre (-74.8997, -35.9997) radius 0.75
  circle A1 centre (-59.5003, -35.9997) radius 0.75
extrude "Extrude18" cut sketch "Sketch10" against normal blind 4.5 contours A0 | A1 bodies 1 in component "Enclosure"
fillet "Fillet1'" radius 1.5 4 edges at (134.4, 20.15, 70.6) (0, 20.15, 70.6) (134.4, 20.15, 0) (0, 20.15, 0) on bodies 1 in component "Enclosure"
sketch "Sketch1 (6)" plane through (0, 40.3, 0) normal (0, 1, 0) x (-1, 0, 0) in component "Back"
  arc A0 (-69.875, 61.85) -> (-68.425, 60.4) centre (-68.425, 61.85) ccw
  line L0 (-65.975, 60.4) -> (-68.425, 60.4)
  arc A1 (-65.975, 60.4) -> (-64.525, 61.85) centre (-65.975, 61.85) ccw
  line L1 (-64.525, 63.35) -> (-64.525, 61.85)
  line L2 (-69.875, 61.85) -> (-69.875, 63.35)
  arc A2 (-68.425, 64.8) -> (-69.875, 63.35) centre (-68.425, 63.35) ccw
  line L3 (-68.425, 64.8) -> (-65.975, 64.8)
  arc A3 (-64.525, 63.35) -> (-65.975, 64.8) centre (-65.975, 63.35) ccw
  line L4 (-131.4, 67.6) -> (-3, 67.6)
  line L5 (-3, 67.6) -> (-3, 3)
  line L6 (-3, 3) -> (-131.4, 3)
  line L7 (-131.4, 3) -> (-131.4, 67.6)
  circle A4 centre (-128.9, 65.1) radius 1.4 construction
  circle A5 centre (-102.518, 64.218) radius 1.5 construction
  circle A6 centre (-31.882, 64.218) radius 1.5 construction
  circle A7 centre (-5.5, 65.1) radius 1.4 construction
  circle A8 centre (-5.5, 5.5) radius 1.4 construction
  circle A9 centre (-128.9, 5.5) radius 1.4 construction
  circle A10 centre (-102.518, 6.382) radius 1.5 construction
  circle A11 centre (-31.882, 6.382) radius 1.5 construction
  circle A12 centre (-128.9, 65.1) radius 1
  circle A13 centre (-102.518, 64.218) radius 1
  circle A14 centre (-31.882, 64.218) radius 1
  circle A15 centre (-5.5, 65.1) radius 1
  circle A16 centre (-5.5, 5.5) radius 1
  circle A17 centre (-31.882, 6.382) radius 1
  circle A18 centre (-102.518, 6.382) radius 1
  arc A19 (-62.7, 9.8) -> (-63.7, 10.8) centre (-63.7, 9.8) ccw construction
  line L8 (-63.7, 10.8) -> (-70.7, 10.8) construction
  arc A20 (-70.7, 10.8) -> (-71.7, 9.8) centre (-70.7, 9.8) ccw construction
  line L9 (-71.7, 9.8) -> (-71.7, 8.6) construction
  arc A21 (-71.7, 8.6) -> (-70.7, 7.6) centre (-70.7, 8.6) ccw construction
  line L10 (-70.7, 7.6) -> (-63.7, 7.6) construction
  arc A22 (-63.7, 7.6) -> (-62.7, 8.6) centre (-63.7, 8.6) ccw construction
  line L11 (-62.7, 8.6) -> (-62.7, 9.8) construction
  arc A23 (-62.5, 9.8) -> (-63.7, 11) centre (-63.7, 9.8) ccw
  line L12 (-63.7, 11) -> (-70.7, 11)
  arc A24 (-70.7, 11) -> (-71.9, 9.8) centre (-70.7, 9.8) ccw
  line L13 (-71.9, 9.8) -> (-71.9, 8.6)
  arc A25 (-71.9, 8.6) -> (-70.7, 7.4) centre (-70.7, 8.6) ccw
  line L14 (-70.7, 7.4) -> (-63.7, 7.4)
  arc A26 (-63.7, 7.4) -> (-62.5, 8.6) centre (-63.7, 8.6) ccw
  line L15 (-62.5, 8.6) -> (-62.5, 9.8)
  circle A27 centre (-128.9, 5.5) radius 1
  point P0 (-131.4, 67.6)
  point P1 (-3, 3)
  dimension "d187" = 2
  dimension "d188" = 2
  dimension "d189" = 2
  dimension "d190" = 2
  dimension "d191" = 2
  dimension "d192" = 2
  dimension "d193" = 2
  dimension "d194" = 0.2
  dimension "d195" = 2
  constraint horizontal L4
  constraint vertical L5
  constraint horizontal L6
  constraint vertical L7
  constraint coincident P1 L5.end
  constraint coincident P0 L4.start
  constraint concentric A4 A12
  constraint concentric A5 A13
  constraint concentric A6 A14
  constraint concentric A7 A15
  constraint concentric A8 A16
  constraint concentric A11 A17
  constraint concentric A10 A18
  constraint concentric A9 A27
  measures "d187" diameter of A12
  measures "d188" diameter of A13
  measures "d189" diameter of A14
  measures "d190" diameter of A15
  measures "d191" diameter of A16
  measures "d192" diameter of A17
  measures "d193" diameter of A18
  measures "d195" diameter of A27
extrude "Extrude1'''''" add sketch "Sketch1 (6)" against normal blind 1.8 separate body contours L4 L5 L6 L7 | A12 | A15 | A16 | A27 makes body 8 in component "Back"
chamfer "Chamfer1'" distance 1.2 angle 45 4 edges at (103.4503, 40.3, 64.5796) (32.8143, 40.3, 64.5796) (32.8143, 40.3, 6.7436) (103.4503, 40.3, 6.7436) on bodies 8 in component "Back"
move_face "OffsetFaces1" offset -0.2 2 faces at (92.7, 18.6333, 64.0667) (105.7, 18.6333, 64.0667) on bodies 3 in component "DisplayMount"
move_face "OffsetFaces2" offset -0.2 2 faces at (28.7, 18.6333, 64.0667) (41.7, 18.6333, 64.0667) on bodies 4 in component "DisplayMount"
move_face "OffsetFaces1'" offset -0.1 4 faces at (131.4, 39.7, 24.5333) (3, 39.7, 46.0667) (45.8, 39.1, 67.6) (88.6, 39.1, 3) on bodies 8 in component "Back"
sketch "Sketch1 (7)" plane through (0, 0, 0) normal (0, -1, 0) x (1, 0, 0) in component "FrontGlass"
  line L0 (2, 68.6) -> (132.4, 68.6)
  line L1 (132.4, 68.6) -> (132.4, 2)
  line L2 (132.4, 2) -> (2, 2)
  line L3 (2, 2) -> (2, 68.6)
  arc A0 (0, 1.5) -> (1.5, 0) centre (1.5, 1.5) ccw
  line L4 (1.5, 0) -> (132.9, 0)
  arc A1 (132.9, 0) -> (134.4, 1.5) centre (132.9, 1.5) ccw
  line L5 (134.4, 1.5) -> (134.4, 69.1)
  arc A2 (134.4, 69.1) -> (132.9, 70.6) centre (132.9, 69.1) ccw
  line L6 (132.9, 70.6) -> (1.5, 70.6)
  arc A3 (1.5, 70.6) -> (0, 69.1) centre (1.5, 69.1) ccw
  line L7 (0, 69.1) -> (0, 1.5)
  line L8 (2, 68.6) -> (132.4, 68.6)
  line L9 (132.4, 68.6) -> (132.4, 2)
  line L10 (132.4, 2) -> (2, 2)
  line L11 (2, 2) -> (2, 68.6)
  constraint horizontal L8
  constraint vertical L9
  constraint horizontal L10
  constraint vertical L11
  constraint coincident L1.end L2.start
  constraint coincident L0.start L3.end
extrude "Extrude1''''''" add sketch "Sketch1 (7)" against normal blind 2.4 separate body contours L0 L1 L2 L3 L8 L9 L10 L11 makes body 9 in component "FrontGlass"
move_face "OffsetFaces3" offset -0.1 4 faces at (101.3, 30.7667, 67.4) (97.1, 30.7667, 3.2) (33.1, 23.0333, 67.4) (37.3, 23.0333, 3.2) on bodies 3 4 in component "DisplayMount"
move_face "OffsetFaces2'" offset -0.2 16 faces at (128.8651, 38.5, 67.232) (106.7, 38.5, 65.6) (91.7, 38.5, 66.6) (66.7917, 38.5, 66.6667) (42.7, 38.5, 66.6) (27.7, 38.5, 66.6) (5.4651, 38.5, 67.232) (5.4651, 38.5, 7.632) (26.7, 38.5, 4) (42.7, 38.5, 4) (3.5, 38.5, 34.3) (63.8, 38.5, 4) (90.7, 38.5, 5) (106.7, 38.5, 5) (128.8651, 38.5, 7.632) (130.4, 38.5, 34.3) on bodies 1 in component "Enclosure"
move_face "OffsetFaces4" offset -0.2 4 faces at (95.1245, 38.5, 65.3667) (95.1245, 38.5, 5.2333) (39.2755, 38.5, 65.3667) (39.2755, 38.5, 5.2333) on bodies 3 4 in component "DisplayMount"
fillet "Fillet1''" radius 0.8 4 edges at (2, 1.2, 68.6) (132.4, 1.2, 68.6) (132.4, 1.2, 2) (2, 1.2, 2) on bodies 9 in component "FrontGlass"
move_face "OffsetFaces2''" offset 0.1 2 faces at (45.7333, 0.8, 68.6) (45.7333, 1.6, 2) on bodies 9 in component "FrontGlass"
sketch "Sketch1 (8)" plane through (0, 0, 0) normal (0, -1, 0) x (1, 0, 0) in component "DXF"
  arc A0 (2, 2.7) -> (2.8, 1.9) centre (2.8, 2.7) ccw
  line L0 (2.8, 1.9) -> (131.6, 1.9)
  arc A1 (131.6, 1.9) -> (132.4, 2.7) centre (131.6, 2.7) ccw
  line L1 (132.4, 2.7) -> (132.4, 67.9)
  arc A2 (132.4, 67.9) -> (131.6, 68.7) centre (131.6, 67.9) ccw
  line L2 (131.6, 68.7) -> (2.8, 68.7)
  arc A3 (2.8, 68.7) -> (2, 67.9) centre (2.8, 67.9) ccw
  line L3 (2, 67.9) -> (2, 2.7)
component "Enclosure" placed x (1, 0, 0) y (0, 1, 0) z (0, 0, 1) at (0, 0, 0)
component "Display" placed x (1, 0, 0) y (0, 1, 0) z (0, 0, 1) at (0, 0, 0)
component "DisplayMount" placed x (1, 0, 0) y (0, 1, 0) z (0, 0, 1) at (0, 0, 0)
component "PwrBoard" placed x (1, 0, 0) y (0, 1, 0) z (0, 0, 1) at (0, 0, 0)
component "LightSensor" placed x (1, 0, 0) y (0, 1, 0) z (0, 0, 1) at (0, 0, 0)
component "Back" placed x (1, 0, 0) y (0, 1, 0) z (0, 0, 1) at (0, 0, 0)
component "FrontGlass" placed x (1, 0, 0) y (0, 1, 0) z (0, 0, 1) at (0, 0, 0)
component "DXF" placed x (1, 0, 0) y (0, 1, 0) z (0, 0, 1) at (0, 0, 0)
equation "dispWidth = 128 mm"
equation "dispHeight = 32.1 mm"
equation "dispThick = 12.9 mm"
equation "wallThick = 3 mm"
equation "frontGlassThick = 2.4 mm"
equation "d6 = dispWidth + wallThick * 2 + tolerance * 2"
equation "d7 = dispHeight * 2 + wallThick * 2 + tolerance * 2"
equation "boardSpaceThick = 25 mm"
equation "d9 = frontGlassThick + dispThick + boardSpaceThick"
equation "d11 = wallThick"
equation "d14 = -frontGlassThick"
equation "d18 = -dispThick"
equation "d37 = wallThick"
equation "d39 = boardSpaceThick - backCoverThick"
equation "backCoverThick = 1.8 mm"
equation "tolerance = 0.2 mm"
equation "d51 = -tolerance"
equation "d59 = wallThick"
equation "d60 = wallThick"
equation "d92 = wallThick"
equation "d93 = wallThick"
equation "d103 = -backCoverThick"
equation "d110 = wallThick"
equation "d111 = wallThick * 2"
equation "pwrBoardLength = 20.4 mm"
equation "pwrBoardWidth = 14 mm"
equation "pwrBoardThick = 1.6 mm"
equation "d123 = wallThick"
equation "d124 = wallThick"
equation "d125 = wallThick"
equation "d126 = wallThick"
equation "d127 = wallThick"
equation "d131 = pwrBoardWidth"
equation "d132 = pwrBoardLength"
equation "d133 = pwrBoardWidth"
equation "d135 = wallThick"
equation "d137 = wallThick + pwrBoardThick"
equation "pwrBoardThickness_1 = 1.6 mm"
equation "d150 = pwrBoardThick"
equation "d160 = 4 mm + wallThick"
equation "d168 = tolerance"
equation "d169 = 4.95 mm + 4 mm"
equation "d170 = 4 mm + wallThick + 2 mm"
equation "d171 = -wallThick"
equation "d179 = -wallThick * 1.5"
equation "d182 = wallThick / 2"
equation "d194 = tolerance"
equation "d196 = -backCoverThick"
equation "d198 = backCoverThick / 1.5"
equation "d199 = wallThick"
equation "d200 = wallThick"
equation "d201 = wallThick"
equation "d202 = wallThick"
equation "d203 = -wallThick"
equation "d205 = wallThick / 2"
equation "d208 = wallThick"
equation "d209 = wallThick"
equation "d212 = -tolerance"
equation "d213 = -tolerance"
equation "d214 = -tolerance / 2"
equation "d215 = -frontGlassThick"
equation "d217 = -tolerance / 2"
equation "d218 = -tolerance"
equation "d219 = -tolerance"
equation "d223 = tolerance * 4"
equation "d226 = tolerance / 2"
named bodies: "Enclosure", "DisplayMountLeft", "DisplayMountRight", "BackCover", "FrontGlass"
